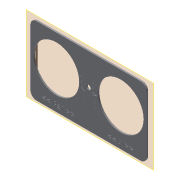
# Autodesk Inventor part: 40_Joystick_PS2_Lid
Saved by Autodesk Inventor 2019.4 (Build 234330000, 330)
## iProperties
Created: 2021-10-05
Part Number: 40_Joystick_PS2_Lid
Material: Generic
Document SubType Name: Modeling
Designer: diederichbenedict
Density: 1 g/cm^3
Appearance: Default
Author: diederichbenedict
Autodesk Inventor part; units mm, degrees
ref_plane "YZ Plane" through (0, 0, 0) normal (1, 0, 0) x (0, 1, 0)
ref_plane "XZ Plane" through (0, 0, 0) normal (0, 1, 0) x (-1, 0, 0)
ref_plane "XY Plane" through (0, 0, 0) normal (0, 0, 1) x (1, 0, 0)
ref_plane "Work Plane1" through (0, 0, 0) normal (0, 0, 1) x (1, 0, 0)
sketch "Sketch1" plane through (0, 0, 0) normal (0, 0, 1) x (1, 0, 0)
  line L0 (36, 18.5) -> (36, -18.5) projected
  arc A0 (34, -20.5) -> (36, -18.5) centre (34, -18.5) ccw projected
  line L1 (34, -20.5) -> (-34, -20.5) projected
  arc A1 (-36, -18.5) -> (-34, -20.5) centre (-34, -18.5) ccw projected
  line L2 (-36, -18.5) -> (-36, 18.5) projected
  arc A2 (-34, 20.5) -> (-36, 18.5) centre (-34, 18.5) ccw projected
  line L3 (-34, 20.5) -> (34, 20.5) projected
  arc A3 (36, 18.5) -> (34, 20.5) centre (34, 18.5) ccw projected
  line L4 (38, -18.5) -> (38, 18.5) projected
  arc A4 (38, 18.5) -> (34, 22.5) centre (34, 18.5) ccw projected
  line L5 (34, 22.5) -> (-34, 22.5) projected
  arc A5 (-34, 22.5) -> (-38, 18.5) centre (-34, 18.5) ccw projected
  line L6 (-38, 18.5) -> (-38, -18.5) projected
  arc A6 (-38, -18.5) -> (-34, -22.5) centre (-34, -18.5) ccw projected
  line L7 (-34, -22.5) -> (34, -22.5) projected
  arc A7 (34, -22.5) -> (38, -18.5) centre (34, -18.5) ccw projected
  circle A8 centre (0, 1.95) radius 1.45 projected
  arc A9 (21.0913, -10.5687) -> (21.0587, 14.5687) centre (21.075, 2) ccw projected
  arc A10 (-21.0587, -10.5687) -> (-21.0913, 14.5687) centre (-21.075, 2) ccw projected
  circle A11 centre (21.075, 2) radius 15
  circle A12 centre (-21.075, 2) radius 15
  point P0 (0, 0)
  dimension "d0" = 30
  dimension "d1" = 30
  constraints: 2 centre point, 2 coincident
  measures "d0" diameter of A11
  measures "d1" diameter of A12
extrude "Extrusion1" add sketch "Sketch1" along normal blind 1 contours L0 A11 A0 L1 A1 L2 A12 A2 L3 A3 | A7 L7 A6 L6 A5 L5 A4 L4
sketch "Sketch2" plane through (0, 0, 0) normal (0, 0, -1) x (-1, 0, 0)
  circle A0 centre (21.075, 2) radius 15 projected
  circle A1 centre (-21.075, 2) radius 15 projected
  circle A2 centre (0, 1.95) radius 1.45 projected
  line L0 (-38, -18.5) -> (-38, 18.5) projected
  arc A3 (-34, 22.5) -> (-38, 18.5) centre (-34, 18.5) ccw projected
  line L1 (-34, 22.5) -> (34, 22.5) projected
  arc A4 (38, 18.5) -> (34, 22.5) centre (34, 18.5) ccw projected
  line L2 (38, 18.5) -> (38, -18.5) projected
  arc A5 (34, -22.5) -> (38, -18.5) centre (34, -18.5) ccw projected
  line L3 (34, -22.5) -> (-34, -22.5) projected
  arc A6 (-38, -18.5) -> (-34, -22.5) centre (-34, -18.5) ccw projected
  line L4 (34, 20.3) -> (-34, 20.3)
  arc A7 (-34, 20.3) -> (-35.8, 18.5) centre (-34, 18.5) ccw
  line L5 (-35.8, 18.5) -> (-35.8, -18.5)
  arc A8 (-35.8, -18.5) -> (-34, -20.3) centre (-34, -18.5) ccw
  line L6 (-34, -20.3) -> (34, -20.3)
  arc A9 (34, -20.3) -> (35.8, -18.5) centre (34, -18.5) ccw
  line L7 (35.8, -18.5) -> (35.8, 18.5)
  arc A10 (35.8, 18.5) -> (34, 20.3) centre (34, 18.5) ccw
  line L8 (-34, 19.8) -> (34, 19.8)
  arc A11 (35.3, 18.5) -> (34, 19.8) centre (34, 18.5) ccw
  line L9 (35.3, 18.5) -> (35.3, -18.5)
  arc A12 (34, -19.8) -> (35.3, -18.5) centre (34, -18.5) ccw
  line L10 (34, -19.8) -> (-34, -19.8)
  arc A13 (-35.3, -18.5) -> (-34, -19.8) centre (-34, -18.5) ccw
  line L11 (-35.3, -18.5) -> (-35.3, 18.5)
  arc A14 (-34, 19.8) -> (-35.3, 18.5) centre (-34, 18.5) ccw
  point P0 (0, 0)
  dimension "d4" = 2.2
  dimension "d5" = 0.5
  constraints: 16 end point, 16 point on circle, 8 centre point, 14 other
  measures "d4" distance between parallel lines of L1 L4
  measures "d5" distance between parallel lines of L4 L8
extrude "Extrusion2" add sketch "Sketch2" along normal blind 1 contours L7 A0 L9 | A0 L9 A11 L8 A14 L11 A1 L5 A7 L4 A10 L7 | L7 A9 L6 A8 L5 A1 L11 A13 L10 A12 L9 A0 | A1 L11 L5
sketch "Sketch3" plane through (0, 0, 1) normal (0, 0, 1) x (1, 0, 0)
  circle A0 centre (-21.075, 2) radius 15 projected
  circle A1 centre (21.075, 2) radius 15 projected
  circle A2 centre (0, 1.95) radius 1.45 projected
  line L0 (38, -18.5) -> (38, 18.5) projected
  arc A3 (38, 18.5) -> (34, 22.5) centre (34, 18.5) ccw projected
  line L1 (34, 22.5) -> (-34, 22.5) projected
  arc A4 (-34, 22.5) -> (-38, 18.5) centre (-34, 18.5) ccw projected
  line L2 (-38, 18.5) -> (-38, -18.5) projected
  arc A5 (-38, -18.5) -> (-34, -22.5) centre (-34, -18.5) ccw projected
  line L3 (-34, -22.5) -> (34, -22.5) projected
  arc A6 (34, -22.5) -> (38, -18.5) centre (34, -18.5) ccw projected
  line L4 (-30.6218, -16.737) -> (-8.9474, -16.737) construction
  line L5 (-8.9474, -16.737) -> (-8.9474, -19.8368) construction
  line L6 (-8.9474, -19.8368) -> (-30.6218, -19.8368) construction
  line L7 (-30.6218, -19.8368) -> (-30.6218, -16.737) construction
  line L8 (-5.485, -9.0267) -> (-5.485, 8.1375) construction
  line L9 (-5.485, 8.1375) -> (-2.437, 8.1375) construction
  line L10 (-2.437, 8.1375) -> (-2.437, -9.0267) construction
  line L11 (-2.437, -9.0267) -> (-5.485, -9.0267) construction
  line L12 (12.255, -17.0504) -> (29.508, -17.0504) construction
  line L13 (29.508, -17.0504) -> (29.508, -20.0984) construction
  line L14 (29.508, -20.0984) -> (12.255, -20.0984) construction
  line L15 (12.255, -20.0984) -> (12.255, -17.0504) construction
  line L16 (2.2253, -8.8386) -> (2.2253, 8.3972) construction
  line L17 (2.2253, 8.3972) -> (5.2733, 8.3972) construction
  line L18 (5.2733, 8.3972) -> (5.2733, -8.8386) construction
  line L19 (5.2733, -8.8386) -> (2.2253, -8.8386) construction
  line L20 (5.1128, -6.2278) -> (4.063, -8.4261)
  line L21 (4.063, -8.4261) -> (3.8185, -8.4261)
  line L22 (3.8185, -8.4261) -> (2.7687, -6.2278)
  line L23 (2.7687, -6.2278) -> (3.1318, -6.2278)
  line L24 (3.1318, -6.2278) -> (3.9395, -7.9321)
  line L25 (3.9395, -7.9321) -> (4.7497, -6.2278)
  line L26 (4.7497, -6.2278) -> (5.1128, -6.2278)
  line L27 (5.1128, -3.1773) -> (4.063, -5.3757)
  line L28 (4.063, -5.3757) -> (3.8185, -5.3757)
  line L29 (3.8185, -5.3757) -> (2.7687, -3.1773)
  line L30 (2.7687, -3.1773) -> (3.1318, -3.1773)
  line L31 (3.1318, -3.1773) -> (3.9395, -4.8817)
  line L32 (3.9395, -4.8817) -> (4.7497, -3.1773)
  line L33 (4.7497, -3.1773) -> (5.1128, -3.1773)
  line L34 (2.2253, 1.0143) -> (3.9247, -0.0157)
  line L35 (3.9247, -0.0157) -> (5.2733, -0.0157)
  line L36 (5.2733, -0.0157) -> (5.2733, -0.4208)
  line L37 (5.2733, -0.4208) -> (3.9667, -0.4208)
  line L38 (3.9667, -0.4208) -> (2.2253, -1.4508)
  line L39 (2.2253, -1.4508) -> (2.2253, -1.0013)
  line L40 (2.2253, -1.0013) -> (3.5665, -0.2158)
  line L41 (3.5665, -0.2158) -> (2.2253, 0.5845)
  line L42 (2.2253, 0.5845) -> (2.2253, 1.0143)
  line L43 (4.063, 4.9342) -> (5.1128, 2.7359)
  line L44 (5.1128, 2.7359) -> (4.7497, 2.7359)
  line L45 (4.7497, 2.7359) -> (3.9395, 4.4402)
  line L46 (3.9395, 4.4402) -> (3.1318, 2.7359)
  line L47 (3.1318, 2.7359) -> (2.7687, 2.7359)
  line L48 (2.7687, 2.7359) -> (3.8185, 4.9342)
  line L49 (3.8185, 4.9342) -> (4.063, 4.9342)
  line L50 (4.063, 7.9847) -> (5.1128, 5.7863)
  line L51 (5.1128, 5.7863) -> (4.7497, 5.7863)
  line L52 (4.7497, 5.7863) -> (3.9395, 7.4907)
  line L53 (3.9395, 7.4907) -> (3.1318, 5.7863)
  line L54 (3.1318, 5.7863) -> (2.7687, 5.7863)
  line L55 (2.7687, 5.7863) -> (3.8185, 7.9847)
  line L56 (3.8185, 7.9847) -> (4.063, 7.9847)
  line L57 (14.8658, -19.9378) -> (12.6675, -18.8881)
  line L58 (12.6675, -18.8881) -> (12.6675, -18.6436)
  line L59 (12.6675, -18.6436) -> (14.8658, -17.5938)
  line L60 (14.8658, -17.5938) -> (14.8658, -17.9569)
  line L61 (14.8658, -17.9569) -> (13.1615, -18.7646)
  line L62 (13.1615, -18.7646) -> (14.8658, -19.5747)
  line L63 (14.8658, -19.5747) -> (14.8658, -19.9378)
  line L64 (17.9162, -19.9378) -> (15.7179, -18.8881)
  line L65 (15.7179, -18.8881) -> (15.7179, -18.6436)
  line L66 (15.7179, -18.6436) -> (17.9162, -17.5938)
  line L67 (17.9162, -17.5938) -> (17.9162, -17.9569)
  line L68 (17.9162, -17.9569) -> (16.2119, -18.7646)
  line L69 (16.2119, -18.7646) -> (17.9162, -19.5747)
  line L70 (17.9162, -19.5747) -> (17.9162, -19.9378)
  line L71 (22.0807, -20.0984) -> (21.6163, -20.0984)
  line L72 (21.6163, -20.0984) -> (20.8753, -18.8831)
  line L73 (20.8753, -18.8831) -> (20.1195, -20.0984)
  line L74 (20.1195, -20.0984) -> (19.6823, -20.0984)
  line L75 (19.6823, -20.0984) -> (20.653, -18.5719)
  line L76 (20.653, -18.5719) -> (19.7119, -17.0504)
  line L77 (19.7119, -17.0504) -> (20.1763, -17.0504)
  line L78 (20.1763, -17.0504) -> (20.9025, -18.2434)
  line L79 (20.9025, -18.2434) -> (21.6435, -17.0504)
  line L80 (21.6435, -17.0504) -> (22.0807, -17.0504)
  line L81 (22.0807, -17.0504) -> (21.1273, -18.5522)
  line L82 (21.1273, -18.5522) -> (22.0807, -20.0984)
  line L83 (26.0451, -18.8881) -> (23.8468, -19.9378)
  line L84 (23.8468, -19.9378) -> (23.8468, -19.5747)
  line L85 (23.8468, -19.5747) -> (25.5511, -18.7646)
  line L86 (25.5511, -18.7646) -> (23.8468, -17.9569)
  line L87 (23.8468, -17.9569) -> (23.8468, -17.5938)
  line L88 (23.8468, -17.5938) -> (26.0451, -18.6436)
  line L89 (26.0451, -18.6436) -> (26.0451, -18.8881)
  line L90 (29.0955, -18.8881) -> (26.8972, -19.9378)
  line L91 (26.8972, -19.9378) -> (26.8972, -19.5747)
  line L92 (26.8972, -19.5747) -> (28.6015, -18.7646)
  line L93 (28.6015, -18.7646) -> (26.8972, -17.9569)
  line L94 (26.8972, -17.9569) -> (26.8972, -17.5938)
  line L95 (26.8972, -17.5938) -> (29.0955, -18.6436)
  line L96 (29.0955, -18.6436) -> (29.0955, -18.8881)
  line L97 (-2.5975, -6.4159) -> (-3.6473, -8.6142)
  line L98 (-3.6473, -8.6142) -> (-3.8918, -8.6142)
  line L99 (-3.8918, -8.6142) -> (-4.9416, -6.4159)
  line L100 (-4.9416, -6.4159) -> (-4.5785, -6.4159)
  line L101 (-4.5785, -6.4159) -> (-3.7708, -8.1202)
  line L102 (-3.7708, -8.1202) -> (-2.9606, -6.4159)
  line L103 (-2.9606, -6.4159) -> (-2.5975, -6.4159)
  line L104 (-2.5975, -3.3654) -> (-3.6473, -5.5637)
  line L105 (-3.6473, -5.5637) -> (-3.8918, -5.5637)
  line L106 (-3.8918, -5.5637) -> (-4.9416, -3.3654)
  line L107 (-4.9416, -3.3654) -> (-4.5785, -3.3654)
  line L108 (-4.5785, -3.3654) -> (-3.7708, -5.0697)
  line L109 (-3.7708, -5.0697) -> (-2.9606, -3.3654)
  line L110 (-2.9606, -3.3654) -> (-2.5975, -3.3654)
  line L111 (-2.437, 0.636) -> (-2.437, -1.4931)
  line L112 (-2.437, -1.4931) -> (-2.8149, -1.4931)
  line L113 (-2.8149, -1.4931) -> (-5.1243, 0.1371)
  line L114 (-5.1243, 0.1371) -> (-5.1243, -1.419)
  line L115 (-5.1243, -1.419) -> (-5.485, -1.419)
  line L116 (-5.485, -1.419) -> (-5.485, 0.594)
  line L117 (-5.485, 0.594) -> (-5.1194, 0.594)
  line L118 (-5.1194, 0.594) -> (-2.7976, -1.0535)
  line L119 (-2.7976, -1.0535) -> (-2.7976, 0.636)
  line L120 (-2.7976, 0.636) -> (-2.437, 0.636)
  line L121 (-3.6473, 4.6745) -> (-2.5975, 2.4762)
  line L122 (-2.5975, 2.4762) -> (-2.9606, 2.4762)
  line L123 (-2.9606, 2.4762) -> (-3.7708, 4.1805)
  line L124 (-3.7708, 4.1805) -> (-4.5785, 2.4762)
  line L125 (-4.5785, 2.4762) -> (-4.9416, 2.4762)
  line L126 (-4.9416, 2.4762) -> (-3.8918, 4.6745)
  line L127 (-3.8918, 4.6745) -> (-3.6473, 4.6745)
  line L128 (-3.6473, 7.725) -> (-2.5975, 5.5267)
  line L129 (-2.5975, 5.5267) -> (-2.9606, 5.5267)
  line L130 (-2.9606, 5.5267) -> (-3.7708, 7.231)
  line L131 (-3.7708, 7.231) -> (-4.5785, 5.5267)
  line L132 (-4.5785, 5.5267) -> (-4.9416, 5.5267)
  line L133 (-4.9416, 5.5267) -> (-3.8918, 7.725)
  line L134 (-3.8918, 7.725) -> (-3.6473, 7.725)
  line L135 (-28.0109, -19.6244) -> (-30.2093, -18.5747)
  line L136 (-30.2093, -18.5747) -> (-30.2093, -18.3301)
  line L137 (-30.2093, -18.3301) -> (-28.0109, -17.2804)
  line L138 (-28.0109, -17.2804) -> (-28.0109, -17.6435)
  line L139 (-28.0109, -17.6435) -> (-29.7153, -18.4512)
  line L140 (-29.7153, -18.4512) -> (-28.0109, -19.2613)
  line L141 (-28.0109, -19.2613) -> (-28.0109, -19.6244)
  line L142 (-24.9605, -19.6244) -> (-27.1588, -18.5747)
  line L143 (-27.1588, -18.5747) -> (-27.1588, -18.3301)
  line L144 (-27.1588, -18.3301) -> (-24.9605, -17.2804)
  line L145 (-24.9605, -17.2804) -> (-24.9605, -17.6435)
  line L146 (-24.9605, -17.6435) -> (-26.6648, -18.4512)
  line L147 (-26.6648, -18.4512) -> (-24.9605, -19.2613)
  line L148 (-24.9605, -19.2613) -> (-24.9605, -19.6244)
  spline S0 degree 2 poles (-20.9763, -17.6558) (-20.9763, -17.8534) (-21.1171, -18.2091) (-21.2431, -18.3326) knots 0 0 0 1 2 2 2
  spline S1 degree 2 poles (-21.2431, -18.3326) (-21.4012, -18.4882) (-21.8285, -18.6488) (-22.1545, -18.6488) knots 0 0 0 1 2 2 2
  line L149 (-22.1545, -18.6488) -> (-22.4979, -18.6488)
  line L150 (-22.4979, -18.6488) -> (-22.4979, -19.785)
  line L151 (-22.4979, -19.785) -> (-22.9029, -19.785)
  line L152 (-22.9029, -19.785) -> (-22.9029, -16.737)
  line L153 (-22.9029, -16.737) -> (-22.1372, -16.737)
  spline S2 degree 2 poles (-22.1372, -16.737) (-21.8655, -16.737) (-21.4852, -16.8259) (-21.3394, -16.9272) knots 0 0 0 1 2 2 2
  spline S3 degree 2 poles (-21.3394, -16.9272) (-21.169, -17.0432) (-20.9763, -17.4014) (-20.9763, -17.6558) knots 0 0 0 1 2 2 2
  spline S4 degree 2 poles (-21.3987, -17.6682) (-21.3987, -17.5101) (-21.5074, -17.2779) (-21.6185, -17.2038) knots 0 0 0 1 2 2 2
  spline S5 degree 2 poles (-21.6185, -17.2038) (-21.7149, -17.1396) (-21.9718, -17.0877) (-22.1619, -17.0877) knots 0 0 0 1 2 2 2
  line L154 (-22.1619, -17.0877) -> (-22.4979, -17.0877)
  line L155 (-22.4979, -17.0877) -> (-22.4979, -18.303)
  line L156 (-22.4979, -18.303) -> (-22.2212, -18.303)
  spline S6 degree 2 poles (-22.2212, -18.303) (-21.9742, -18.303) (-21.6704, -18.2239) (-21.5716, -18.1202) knots 0 0 0 1 2 2 2
  spline S7 degree 2 poles (-21.5716, -18.1202) (-21.4802, -18.0288) (-21.3987, -17.8139) (-21.3987, -17.6682) knots 0 0 0 1 2 2 2
  spline S8 degree 2 poles (-19.6277, -19.8368) (-20.1761, -19.8368) (-20.7787, -19.2218) (-20.7787, -18.6537) knots 0 0 0 1 2 2 2
  spline S9 degree 2 poles (-20.7787, -18.6537) (-20.7787, -18.0955) (-20.1933, -17.4335) (-19.7216, -17.4335) knots 0 0 0 1 2 2 2
  spline S10 degree 2 poles (-19.7216, -17.4335) (-19.5091, -17.4335) (-19.1806, -17.557) (-19.0596, -17.6879) knots 0 0 0 1 2 2 2
  spline S11 degree 2 poles (-19.0596, -17.6879) (-18.9361, -17.8188) (-18.8052, -18.1967) (-18.8052, -18.4709) knots 0 0 0 1 2 2 2
  line L157 (-18.8052, -18.4709) -> (-18.8052, -18.6809)
  line L158 (-18.8052, -18.6809) -> (-20.3885, -18.6809)
  spline S12 degree 2 poles (-20.3885, -18.6809) (-20.3885, -19.0785) (-19.9883, -19.5009) (-19.6326, -19.5009) knots 0 0 0 1 2 2 2
  spline S13 degree 2 poles (-19.6326, -19.5009) (-19.5067, -19.5009) (-19.2621, -19.4441) (-19.1633, -19.3996) knots 0 0 0 1 2 2 2
  spline S14 degree 2 poles (-19.1633, -19.3996) (-19.0596, -19.3502) (-18.9163, -19.2638) (-18.8694, -19.2243) knots 0 0 0 1 2 2 2
  line L159 (-18.8694, -19.2243) -> (-18.8472, -19.2243)
  line L160 (-18.8472, -19.2243) -> (-18.8472, -19.6442)
  spline S15 degree 2 poles (-18.8472, -19.6442) (-18.9139, -19.6713) (-19.1164, -19.7504) (-19.1955, -19.7726) knots 0 0 0 1 2 2 2
  spline S16 degree 2 poles (-19.1955, -19.7726) (-19.3066, -19.8047) (-19.4894, -19.8368) (-19.6277, -19.8368) knots 0 0 0 1 2 2 2
  spline S17 degree 2 poles (-19.1806, -18.3869) (-19.1856, -18.2313) (-19.2498, -18.0041) (-19.3115, -17.9275) knots 0 0 0 1 2 2 2
  spline S18 degree 2 poles (-19.3115, -17.9275) (-19.3782, -17.8411) (-19.5882, -17.7497) (-19.7438, -17.7497) knots 0 0 0 1 2 2 2
  spline S19 degree 2 poles (-19.7438, -17.7497) (-19.8969, -17.7497) (-20.1118, -17.8411) (-20.2008, -17.93) knots 0 0 0 1 2 2 2
  spline S20 degree 2 poles (-20.2008, -17.93) (-20.2872, -18.0214) (-20.3761, -18.2412) (-20.3885, -18.3869) knots 0 0 0 1 2 2 2
  line L161 (-20.3885, -18.3869) -> (-19.1806, -18.3869)
  line L162 (-16.6192, -19.785) -> (-17.0046, -19.785)
  line L163 (-17.0046, -19.785) -> (-17.0046, -18.4808)
  spline S21 degree 2 poles (-17.0046, -18.4808) (-17.0046, -18.3227) (-17.0342, -18.051) (-17.0787, -17.9695) knots 0 0 0 1 2 2 2
  spline S22 degree 2 poles (-17.0787, -17.9695) (-17.1256, -17.8831) (-17.2935, -17.7991) (-17.4368, -17.7991) knots 0 0 0 1 2 2 2
  spline S23 degree 2 poles (-17.4368, -17.7991) (-17.5801, -17.7991) (-17.8839, -17.9522) (-18.0296, -18.0757) knots 0 0 0 1 2 2 2
  line L164 (-18.0296, -18.0757) -> (-18.0296, -19.785)
  line L165 (-18.0296, -19.785) -> (-18.4149, -19.785)
  line L166 (-18.4149, -19.785) -> (-18.4149, -17.4977)
  line L167 (-18.4149, -17.4977) -> (-18.0296, -17.4977)
  line L168 (-18.0296, -17.4977) -> (-18.0296, -17.7521)
  spline S24 degree 2 poles (-18.0296, -17.7521) (-17.8567, -17.5965) (-17.5233, -17.4335) (-17.3355, -17.4335) knots 0 0 0 1 2 2 2
  spline S25 degree 2 poles (-17.3355, -17.4335) (-16.9996, -17.4335) (-16.6192, -17.8781) (-16.6192, -18.3005) knots 0 0 0 1 2 2 2
  line L169 (-16.6192, -18.3005) -> (-16.6192, -19.785)
  line L170 (-12.4103, -18.5747) -> (-14.6086, -19.6244)
  line L171 (-14.6086, -19.6244) -> (-14.6086, -19.2613)
  line L172 (-14.6086, -19.2613) -> (-12.9043, -18.4512)
  line L173 (-12.9043, -18.4512) -> (-14.6086, -17.6435)
  line L174 (-14.6086, -17.6435) -> (-14.6086, -17.2804)
  line L175 (-14.6086, -17.2804) -> (-12.4103, -18.3301)
  line L176 (-12.4103, -18.3301) -> (-12.4103, -18.5747)
  line L177 (-9.3599, -18.5747) -> (-11.5582, -19.6244)
  line L178 (-11.5582, -19.6244) -> (-11.5582, -19.2613)
  line L179 (-11.5582, -19.2613) -> (-9.8539, -18.4512)
  line L180 (-9.8539, -18.4512) -> (-11.5582, -17.6435)
  line L181 (-11.5582, -17.6435) -> (-11.5582, -17.2804)
  line L182 (-11.5582, -17.2804) -> (-9.3599, -18.3301)
  line L183 (-9.3599, -18.3301) -> (-9.3599, -18.5747)
  point P0 (0, 0)
  constraints: 8 other
extrude "Extrusion3" cut sketch "Sketch3" against normal blind 0.5 contours L20 L21 L22 L23 L24 L25 L26 | L27 L28 L29 L30 L31 L32 L33 | L34 L35 L36 L37 L38 L39 L40 L41 L42 | L43 L44 L45 L46 L47 L48 L49 | L50 L51 L52 L53 L54 L55 L56 | L57 L58 L59 L60 L61 L62 L63 | L64 L65 L66 L67 L68 L69 L70 | L71 L72 L73 L74 L75 L76 L77 L78 L79 L80 L81 L82 | L83 L84 L85 L86 L87 L88 L89 | L90 L91 L92 L93 L94 L95 L96 | L97 L98 L99 L100 L101 L102 L103 | L104 L105 L106 L107 L108 L109 L110 | L111 L112 L113 L114 L115 L116 L117 L118 L119 L120 | L121 L122 L123 L124 L125 L126 L127 | L128 L129 L130 L131 L132 L133 L134 | L135 L136 L137 L138 L139 L140 L141 | L142 L143 L144 L145 L146 L147 L148 | S0 S1 L149 L150 L151 L152 L153 S2 S3 | S8 S9 S10 S11 L157 L158 S12 S13 S14 L159 L160 S15 S16 | L162 L163 S21 S22 S23 L164 L165 L166 L167 L168 S24 S25 L169 | L170 L171 L172 L173 L174 L175 L176 | L177 L178 L179 L180 L181 L182 L183
body "Solid1"
